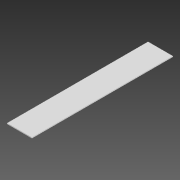
# Autodesk Inventor part: border1
Saved by Autodesk Inventor 2020 (Build 240168000, 168)
## iProperties
Created: 2022-08-25
Part Number: border1
Material: Generic
Document SubType Name: Modeling
Designer: Umair
Density: 1 g/cm^3
Appearance: Default
Author: Umair
Autodesk Inventor part; units mm, degrees
ref_plane "YZ Plane" through (0, 0, 0) normal (1, 0, 0) x (0, 1, 0)
ref_plane "XZ Plane" through (0, 0, 0) normal (0, 1, 0) x (-1, 0, 0)
ref_plane "XY Plane" through (0, 0, 0) normal (0, 0, 1) x (1, 0, 0)
sketch "Sketch1" plane through (0, 0, 0) normal (0, 1, 0) x (-1, 0, 0)
  line L0 (55, 312.5) -> (-55, 312.5)
  line L1 (-55, 312.5) -> (-55, -312.5)
  line L2 (-55, -312.5) -> (55, -312.5)
  line L3 (55, -312.5) -> (55, 312.5)
  line L4 (55, 312.5) -> (-55, -312.5) construction
  line L5 (-55, 312.5) -> (55, -312.5) construction
  point P0 (0, 0)
  dimension "d0" = 110
  dimension "d1" = 625
  constraints: 12 end point, 2 midpoint, 2 parallel, 1 horizontal, 1 perpendicular
  measures "d0" distance of L2.end L1.end
  measures "d1" distance of L1.end L0.end
extrude "Extrusion1" add sketch "Sketch1" along normal blind 3
body "Solid1"
